Couch Foot (Autodesk Fusion 360 design; units mm, degrees)
Autodesk Fusion 360 part; units mm, degrees
sketch "Couch Foot Base" plane through (0, 0, 0) normal (0, 0, 1) x (1, 0, 0) in component "Couch Foot"
  circle A0 centre (0, 0) radius 16.5
  circle A1 centre (0, 0) radius 9
  circle A2 centre (0, 0) radius 3.5
  dimension "d4" = 18
  dimension "d5" = 33
  dimension "d6" = 7
  constraint coincident A0.centre A1.centre
  constraint concentric A0 A1
  measures "d4" diameter of A1
  measures "d5" diameter of A0
  measures "d6" diameter of A2
extrude "Extrude1" add sketch "Couch Foot Base" along normal blind 12 contours A0 makes body 1 in component "Couch Foot"
extrude "Extrude2" add sketch "Couch Foot Base" along normal blind 4 contours A1 bodies 1 in component "Couch Foot"
draft "Draft1" angle -3 neutral plane through (0, 0, 0) pull (0, 0, -1) 1 faces at (16.4795, -0.8225, 8) on bodies 1 in component "Couch Foot"
draft "Draft2" angle -3 neutral plane through (0, 0, 0) pull (0, 0, -1) 1 faces at (8.9553, -0.8961, 9.3333) on bodies 1 in component "Couch Foot"
chamfer "Chamfer1" distance 1 angle 45 3 edges at (-14.7971, -5.7392, 12) (-8.9773, 3.482, 12) (-3.2631, 1.2657, 4) on bodies 1 in component "Couch Foot"
box "BoxPrimitive1" add length 200 width 200 height -10 placed x (0, -1, 0) y (1, 0, 0) z (0, 0, 1) at (-113.8921, 61.0069, 0) separate body makes body 2 in component "Table for Render"
component "Couch Foot" placed x (1, 0, 0) y (0, 1, 0) z (0, 0, 1) at (0, 0, 0)
component "Table for Render" placed x (1, 0, 0) y (0, 1, 0) z (0, 0, 1) at (0, 0, 0)
named bodies: "Couch Foot", "Table"
